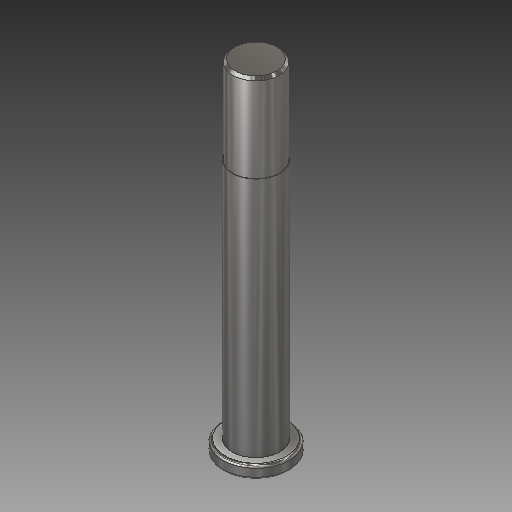
# Autodesk Inventor part: paris_kingpin
Saved by Autodesk Inventor 2019.3 (Build 233278000, 278)
## iProperties
Created: 2017-04-02
Part Number: paris_kingpin
Material: Типовые
Document SubType Name: Modeling
Designer: Nikita
Density: 1 g/cm^3
Appearance: Сталь — полированная
Mass: 4.62241 g
Surface Area: 22.0031 cm^2
Volume: 4.62241 cm^3
Author: Nikita
Autodesk Inventor part; units mm, degrees
ref_plane "YZ Plane" through (0, 0, 0) normal (1, 0, 0) x (0, 1, 0)
ref_plane "XZ Plane" through (0, 0, 0) normal (0, 1, 0) x (-1, 0, 0)
ref_plane "XY Plane" through (0, 0, 0) normal (0, 0, 1) x (1, 0, 0)
sketch "Эскиз1" plane through (0, 0, 0) normal (0, 0, 1) x (1, 0, 0)
  line L0 (0, 0) -> (6.5, 0)
  line L1 (6.5, 0) -> (6.5, 2.5)
  line L2 (6.5, 2.5) -> (4.65, 2.5)
  line L3 (4.65, 2.5) -> (4.65, 49.5)
  line L4 (4.65, 49.5) -> (4.55, 49.5)
  line L5 (4.55, 49.5) -> (4.55, 66.5)
  line L6 (4.55, 66.5) -> (0, 66.5)
  line L7 (0, 66.5) -> (0, 0)
  dimension "d1" = 64
  dimension "d2" = 9.3
  dimension "d3" = 0.1
  dimension "d4" = 13
  dimension "d5" = 2.5
  dimension "d6" = 17
  constraints: 16 end point, 7 perpendicular, 1 horizontal
  measures "d1" distance between parallel lines of L2 L6
  measures "d2" diameter of L3 L7
  measures "d3" distance between parallel lines of L3 L5
  measures "d4" diameter of L1 L7
  measures "d5" distance of L0.end L1.end
  measures "d6" distance of L4.end L5.end
revolve "Вращение1" add sketch "Эскиз1" angle 360 about axis through (0, 66.5, 0) along (0, -1, 0)
fillet "Сопряжение1" radius 0.5 2 edges at (-6.5, 2.5, 0) (-6.5, 0, 0)
chamfer "Фаска1" distance 0.5 angle 45 1 edges at (-4.55, 66.5, 0)
